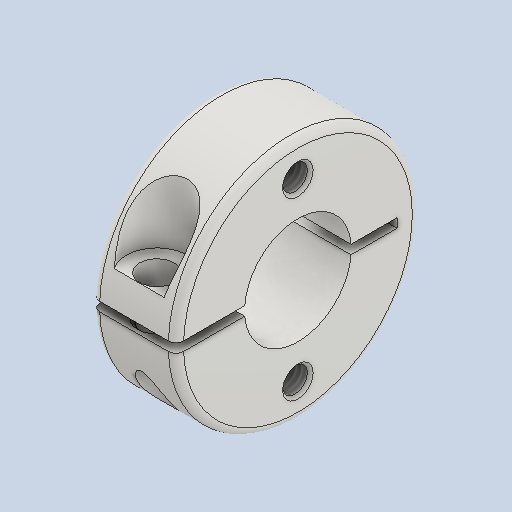
# Autodesk Inventor part: 62311400GA_1
Saved by Autodesk Inventor 2025.4 (Build 294407000, 407)
## iProperties
Category: PARTsolutions
Company: MAEDLER
Created: 2026-04-27
Part Number: 62311400GA_1
Material: Steel AISI 1045 225 ANLD
Catalog Web Link: www.3dfindit.com
Description: geschl_klr_typ_ga-Round body, Shaft Collars, Clamp Collars, Single-Split - Type GA, Diameter 10mm - 50mm, Material steel burnished and stainless steel 1.4305
Vendor: MAEDLER
Document SubType Name: Modeling
Designer: psAdmin
Manufacturer: MAEDLER
Mass: 49.7731 g
Surface Area: 34.1886 cm^2
Volume: 6.34052 cm^3
Density: 7.85 g/cm^3
Appearance: Steel
PSOL_IDENT_0: {$CADENAS_DATA/23d-libs/maedler/antriebselemente/klemmringe_stellringe/klemmringe/geschl_klemmringe_
PSOL_IDENT_1: ausf_ga/geschl_klr_typ_ga.prj},175 {VTYP=3D},{NB=62311400GA_1},{LINA=62311400GA},{NN=geschl_klr_typ_
PSOL_IDENT_2: ga},{DATE=23.11.2024 12:14:57},{GEOMDATE=04.08.2024 13:07:05},{VERSION=},{LINEID=2670},{WBVAR=},{WBN
PSOL_IDENT_3: UMERIC=}  {NB=62311400GA_1},{LINA=62311400GA},{KT=DUMMY},{ARTNR=62311400GA},{WEBSHOP=Produktdetails
PSOL_IDENT_4: / Katalogseite / Montageanleitung},{MATK=Stahl},{MAT=Stahl C45 brüniert, Schraube mit Festigkeit 12.
PSOL_IDENT_5: 9},{D1=14},{D2=32},{R=33.9},{B=11},{SDIN912=M4 x 14},{M=23.0},{G=M4},{GEW=49},{GG=4},{A=13.0},{T=4.0
PSOL_IDENT_6: },{H=4.5},{J=8},{D3=3.24},{D4=4},{F1=1},{S=1.2},{TN=geschl_klr_typ_ga_st_14},{CTN=84839089},{DIST=2.
PSOL_IDENT_7: 15},{CNSDWTEMPLATE=_dw/ansicht_front_left.dw}
NB: 62311400GA_1
NN: geschl_klr_typ_ga
NT: Round body, Shaft Collars, Clamp Collars, Single-Split - Type GA, Diameter 10mm - 50mm, Material steel burnished and stainless steel 1.4305
NBSYN: $ARTNR._1
LINA: 62311400GA
CATALOG: MÄDLER
ARTNR: 62311400GA
WEBSHOP: Product details / Catalogue page / Assembly instructions
MATK: Steel
MAT: Steel C45 black oxide finish, Screw with strength 12.9
D1: 14
D2: 32
R: 33.9
B: 11
SDIN912: M4 x 14
M: 23
G: M4
GEW: 49
GG: 4
A: 13
T: 4
H: 4.5
J: 8
D3: 3.24
D4: 4
F1: 1
S: 1.2
TN: geschl_klr_typ_ga_st_14
CTN: 84839089
SUPPLIER: MAEDLER
ARTICLENO: 62311400GA_1
BOMINFO: 62311400GA
CREATOR: CADENAS GmbH
Title: 62311400GA
Author: Cadenas PARTsolutions
Comments: Round body, Shaft Collars, Clamp Collars, Single-Split - Type GA, Diameter 10mm - 50mm, Material steel burnished and stainless steel 1.4305
Autodesk Inventor part; units mm, degrees
sketch "Skizze_1" plane through (0, 0, 0) normal (0, 0, 1) x (1, 0, 0)
  line L0 (5.5, 0) -> (-5.5, 0)
  line L1 (-5.5, 15) -> (-5.5, 7)
  line L2 (-5.5, 7) -> (5.5, 7)
  line L3 (5.5, 7) -> (5.5, 15)
  arc A0 (5.5, 15) -> (4.5, 16) centre (4.5, 15) ccw
  line L4 (4.5, 16) -> (-4.5, 16)
  arc A1 (-4.5, 16) -> (-5.5, 15) centre (-4.5, 15) ccw
  constraints: 10 end point, 4 point on circle, 2 centre point
revolve "Revolution1" add sketch "Skizze_1" angle 360 about axis through (5.5, 0, 0) along (1, 0, 0)
sketch "Sketch_4" plane through (0, 0, 0) normal (1, 0, 0) x (0, 0, -1)
  line L0 (-21, 0.6) -> (-21, -0.6)
  line L1 (-21, -0.6) -> (13, -0.6)
  line L2 (13, -0.6) -> (13, 0.6)
  line L3 (13, 0.6) -> (-21, 0.6)
  constraints: 8 end point
extrude "Extrusion1" cut sketch "Sketch_4" along normal mid plane 22
sketch "Sketch_6" plane through (0, 0, 13) normal (0, 0, 1) x (1, 0, 0)
  line L0 (0, 0) -> (0, 21)
  line L1 (0, 21) -> (4, 21)
  line L2 (4, 21) -> (4, 4.6)
  line L3 (4, 4.6) -> (2.25, 4.6)
  line L4 (2.25, 4.6) -> (2.25, 0)
  line L5 (2.25, 0) -> (0, 0)
  line L6 (0, 0) -> (0, 21)
  constraints: 14 end point
revolve "Revolution2" cut sketch "Sketch_6" angle 360 about axis through (0, 0, 13) along (0, -1, 0)
sketch "Sketch_2" plane through (0, 11.5, 0) normal (0, 1, 0) x (1, 0, 0)
  line L0 (5.5, 0) -> (-5.5, 0)
  line L1 (-5.5, 0) -> (-5.5, 2)
  line L2 (-5.5, 2) -> (-5.121, 1.621)
  line L3 (-5.121, 1.621) -> (5.121, 1.621)
  line L4 (5.121, 1.621) -> (5.5, 2)
  line L5 (5.5, 2) -> (5.5, 0)
  line L6 (5.5, 0) -> (-5.5, 0)
  constraints: 14 end point
revolve "Revolution3" cut sketch "Sketch_2" angle 360 about axis through (5.5, 11.5, 0) along (1, 0, 0)
thread "Thread1" size "M4x0.7" class "6H" standard "ISO Metric profile" full length
sketch "Sketch_3" plane through (0, -11.5, 0) normal (0, 1, 0) x (1, 0, 0)
  line L0 (5.5, 0) -> (-5.5, 0)
  line L1 (-5.5, 0) -> (-5.5, 2)
  line L2 (-5.5, 2) -> (-5.121, 1.621)
  line L3 (-5.121, 1.621) -> (5.121, 1.621)
  line L4 (5.121, 1.621) -> (5.5, 2)
  line L5 (5.5, 2) -> (5.5, 0)
  line L6 (5.5, 0) -> (-5.5, 0)
  constraints: 14 end point
revolve "Revolution4" cut sketch "Sketch_3" angle 360 about axis through (5.5, -11.5, 0) along (1, 0, 0)
thread "Thread2" size "M4x0.7" class "6H" standard "ISO Metric profile" full length
sketch "Sketch_1" plane through (0, 0, 0) normal (1, 0, 0) x (0, 0, -1)
  line L0 (-13, -9.5555) -> (-13, -0.6)
  line L1 (-13, -0.6) -> (-10.5, -0.6)
  line L2 (-10.5, -0.6) -> (-11, -1.1)
  line L3 (-11, -1.1) -> (-11, -11.8471)
  line L4 (-11, -11.8471) -> (-13, -9.5555)
  line L5 (-13, -9.5555) -> (-13, -0.6)
  constraints: 12 end point
revolve "Revolution5" cut sketch "Sketch_1" angle 360 about axis through (0, -9.5555, 13) along (0, -1, 0)
ref_plane "D2X1_XY" through (5.5, 16, 0) normal (0, 0, 1) x (1, 0, 0)
ref_plane "D2X1_YZ" through (5.5, 16, 0) normal (1, 0, 0) x (0, 1, 0)
ref_plane "D2X1_ZX" through (5.5, 16, 0) normal (0, 1, 0) x (0, 0, 1)
ref_plane "D2X2_XY" through (5.5, -16, 0) normal (0, 0, 1) x (1, 0, 0)
ref_plane "D2X2_YZ" through (5.5, -16, 0) normal (1, 0, 0) x (0, 1, 0)
ref_plane "D2X2_ZX" through (5.5, -16, 0) normal (0, 1, 0) x (0, 0, 1)
ref_plane "schraubenkopf_XY" through (0, 4.6, 13) normal (0, 1, 0) x (1, 0, 0)
ref_plane "schraubenkopf_YZ" through (0, 4.6, 13) normal (1, 0, 0) x (0, 0, -1)
ref_plane "schraubenkopf_ZX" through (0, 4.6, 13) normal (0, 0, -1) x (0, 1, 0)
body "Solid1"
